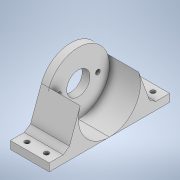
# Autodesk Inventor part: motor mount
Saved by Autodesk Inventor 2020.3 (Build 243373000, 373)
## iProperties
Created: 2020-08-10
Part Number: motor mount
Material: Generic
Document SubType Name: Modeling
Designer: joesp
Density: 1 g/cm^3
Appearance: Default
Author: joesp
Autodesk Inventor part; units mm, degrees
ref_plane "YZ Plane" through (0, 0, 0) normal (1, 0, 0) x (0, 1, 0)
ref_plane "XZ Plane" through (0, 0, 0) normal (0, 1, 0) x (-1, 0, 0)
ref_plane "XY Plane" through (0, 0, 0) normal (0, 0, 1) x (1, 0, 0)
sketch "Sketch1" plane through (0, 0, 0) normal (1, 0, 0) x (0, 1, 0)
  arc A0 (26.8706, 20) -> (26.8706, 57.5657) centre (20, 38.7829) ccw
  line L0 (5, 77.5657) -> (0, 77.5657)
  line L1 (0, 77.5657) -> (0, 0)
  line L2 (0, 0) -> (5, 0)
  circle A1 centre (20, 38.7829) radius 20 construction
  circle A2 centre (20, 26.2829) radius 1.5
  circle A3 centre (20, 51.2829) radius 1.5
  circle A4 centre (20, 38.7829) radius 7.5
  line L3 (26.8706, 57.5657) -> (5, 65.5657)
  line L4 (5, 65.5657) -> (5, 77.5657)
  line L5 (26.8706, 20) -> (5, 12)
  line L6 (5, 12) -> (5, 0)
  dimension "d0" = 20
  dimension "d1" = 20
  dimension "d3" = 5
  dimension "d5" = 3
  dimension "d6" = 3
  dimension "d7" = 25
  dimension "d8" = 12.5
  dimension "d9" = 15
  dimension "d12" = 20
  dimension "d13" = 12
  constraints: 14 end point, 5 centre point, 4 coincident, 4 point on circle, 4 vertical alignment, 3 tangent, 2 perpendicular, 1 collinear, 1 concentric, 1 horizontal, 1 point on line, 1 vertical
  measures "d0" radius of A0
  measures "d1" vertical distance of L3.start L0.end
  measures "d3" distance of L0.start L0.end
  measures "d5" diameter of A3
  measures "d6" diameter of A2
  measures "d7" distance of A2.centre A3.centre
  measures "d8" distance of point (20, 38.783) A2.centre
  measures "d9" diameter of A4
  measures "d12" distance from line of L2 L5.start
  measures "d13" distance of L3.end L0.start
extrude "Extrusion1" add sketch "Sketch1" along normal blind 5
sketch "Sketch2" plane through (5, 0, 0) normal (1, 0, 0) x (0, 0, -1)
  line L0 (-77.5657, 5) -> (-77.5657, 0) projected
  line L1 (-57.5657, 26.8706) -> (-65.5657, 5) projected
  line L2 (-77.5657, 5) -> (-65.5657, 5)
  line L3 (-65.5657, 5) -> (-57.5657, 26.8706)
  line L4 (-77.5657, 0) -> (0, 0) projected
  line L5 (-77.5657, 0) -> (0, 0)
  line L6 (-77.5657, 0) -> (-77.5657, 5)
  circle A0 centre (-38.7829, 20) radius 20
  arc A1 (-20, 26.8706) -> (-57.5657, 26.8706) centre (-38.7829, 20) ccw projected
  line L7 (0, 0) -> (0, 5) projected
  line L8 (0, 0) -> (0, 5)
  line L9 (0, 5) -> (-12, 5)
  line L10 (-12, 5) -> (-20, 26.8706) projected
  line L11 (-12, 5) -> (-20, 26.8706)
  point P0 (-20, 26.8706)
  point P1 (-38.7829, 0)
  constraints: 14 end point, 3 collinear, 2 perpendicular, 1 coincident, 1 horizontal, 1 vertical, 5 other
extrude "Extrusion2" add sketch "Sketch2" along normal blind 20 contours L2 L1 A0 L4 L0 | A0 L10 L9 L7 L4
chamfer "Chamfer1" distance 3 angle 45 2 edges at (12.5, 5, 12) (12.5, 5, 65.5657)
sketch "Sketch3" plane through (0, 5, 0) normal (0, 1, 0) x (1, 0, 0)
  circle A0 centre (6.25, -4.5) radius 1.5
  circle A1 centre (18.75, -4.5) radius 1.5
  circle A2 centre (6.25, -73.0657) radius 1.5
  circle A3 centre (18.75, -73.0657) radius 1.5
  line L0 (0, -77.5657) -> (25, -77.5657) projected
  line L1 (0, -68.5657) -> (25, -68.5657) projected
  line L2 (0, 0) -> (25, 0) projected
  line L3 (25, -9) -> (0, -9) projected
  line L4 (0, -68.5657) -> (0, -77.5657) projected
  line L5 (25, -68.5657) -> (25, -77.5657) projected
  dimension "d20" = 3
  dimension "d21" = 4.5
  dimension "d22" = 4.5
  dimension "d23" = 4.5
  dimension "d24" = 4.5
  dimension "d25" = 6.25
  dimension "d26" = 6.25
  dimension "d27" = 12.5
  constraints: 4 centre point, 3 equal radius, 2 horizontal alignment, 2 vertical alignment
  measures "d20" diameter of A2
  measures "d21" distance from line of L0 A2.centre
  measures "d22" distance from line of L1 A2.centre
  measures "d23" distance from line of L2 A0.centre
  measures "d24" distance from line of L3 A0.centre
  measures "d25" distance from line of L4 A2.centre
  measures "d26" distance from line of L5 A3.centre
  measures "d27" distance of A2.centre A3.centre
extrude "Extrusion3" cut sketch "Sketch3" against normal through all contours A0 | A1 | A2 | A3
equation "\"d8\" = 0.5 * d7"
equation "\"d12\" = d1"
equation "\"d21\" = d22"
equation "\"d23\" = d24"
equation "\"d25\" = 0.5 * d27"
equation "\"d26\" = d25"
body "Solid1"
